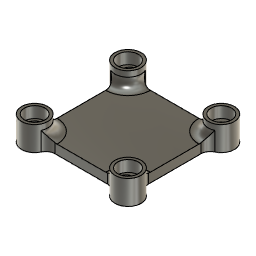
base (Autodesk Fusion 360 design; units mm, degrees)
Autodesk Fusion 360 part; units mm, degrees
sketch "Sketch1" plane through (0, 0, 0) normal (0, 0, 1) x (1, 0, 0)
  line L0 (-25, 25) -> (25, 25) construction
  line L1 (25, 25) -> (25, -25) construction
  line L2 (25, -25) -> (-25, -25) construction
  line L3 (-25, -25) -> (-25, 25) construction
  circle A0 centre (-25, 25) radius 7
  circle A1 centre (25, 25) radius 3.25
  circle A2 centre (25, -25) radius 7
  circle A3 centre (-25, -25) radius 4
  circle A4 centre (-25, -25) radius 7
  circle A5 centre (25, 25) radius 7
  line L4 (-28.25, 26) -> (-28.25, 24)
  arc A6 (-28.25, 24) -> (-21.75, 24) centre (-25, 24) ccw
  line L5 (-21.75, 24) -> (-21.75, 26)
  arc A7 (-21.75, 26) -> (-28.25, 26) centre (-25, 26) ccw
  line L6 (-25, 26) -> (-25, 24) construction
  line L7 (24, -28.25) -> (26, -28.25)
  arc A8 (26, -28.25) -> (26, -21.75) centre (26, -25) ccw
  line L8 (26, -21.75) -> (24, -21.75)
  arc A9 (24, -21.75) -> (24, -28.25) centre (24, -25) ccw
  line L9 (24, -25) -> (26, -25) construction
  line L10 (-18, 25) -> (18, 25)
  line L11 (25, 18) -> (25, -18)
  line L12 (18, -25) -> (-18, -25)
  line L13 (-25, -18) -> (-25, 18)
  circle A10 centre (-25, 25) radius 5.5
  circle A11 centre (25, 25) radius 5.5
  circle A12 centre (-25, -25) radius 5.5
  circle A13 centre (25, -25) radius 5.5
  line L14 (-7, 10) -> (-3, 10)
  line L15 (-3, 10) -> (-3, -10)
  line L16 (-3, -10) -> (-7, -10)
  line L17 (-7, -10) -> (-7, 10)
  line L18 (3, 10) -> (7, 10)
  line L19 (7, 10) -> (7, -10)
  line L20 (7, -10) -> (3, -10)
  line L21 (3, -10) -> (3, 10)
  point P0 (-25, 25)
  point P1 (25, -25)
  dimension "d1" = 50
  dimension "d2" = 50
  dimension "d3" = 25
  dimension "d4" = 25
  dimension "d5" = 6.5
  dimension "d6" = 14
  dimension "d7" = 8
  dimension "d8" = 14
  dimension "d9" = 14
  dimension "d10" = 14
  dimension "d11" = 6.5
  dimension "d12" = 2
  dimension "d13" = 6.5
  dimension "d14" = 2
  dimension "d17" = 11
  dimension "d18" = 11
  dimension "d19" = 11
  dimension "d20" = 11
  dimension "d27" = 3
  dimension "d28" = 3
  dimension "d29" = 4
  dimension "d30" = 4
  dimension "d31" = 20
  dimension "d32" = 20
  dimension "d33" = 10
  dimension "d34" = 10
  constraint horizontal L0
  constraint vertical L1
  constraint horizontal L2
  constraint vertical L3
  constraint coincident P0 L0.start
  constraint coincident L0.end L1.start
  constraint coincident P1 L1.end
  constraint coincident L2.end L3.start
  constraint concentric A3 A4
  constraint concentric A1 A5
  constraint tangent L4 A6
  constraint tangent A6 L5
  constraint parallel L4 L5
  constraint tangent L5 A7
  constraint tangent L4 A7
  constraint coincident L3 A6.centre
  constraint perpendicular L0 L6
  constraint midpoint L6 P0
  constraint tangent L7 A8
  constraint tangent A8 L8
  constraint parallel L7 L8
  constraint tangent L8 A9
  constraint tangent L7 A9
  constraint perpendicular L1 L9
  constraint midpoint L9 P1
  constraint coincident A0 L10.start
  constraint coincident L0 L10.start
  constraint coincident A5 L10.end
  constraint coincident L0 L10.end
  constraint coincident L1 L11.start
  constraint coincident A5 L11.start
  constraint coincident A2 L11.end
  constraint coincident L1 L11.end
  constraint coincident A2 L12.start
  constraint coincident L2 L12.start
  constraint coincident A4 L12.end
  constraint coincident L2 L12.end
  constraint coincident A4 L13.start
  constraint coincident L3 L13.start
  constraint coincident L3 L13.end
  constraint coincident A0 L13.end
  constraint concentric A5 A11
  constraint concentric A4 A12
  constraint horizontal L14
  constraint vertical L15
  constraint horizontal L16
  constraint vertical L17
  constraint horizontal L18
  constraint vertical L19
  constraint horizontal L20
  constraint vertical L21
  measures "d1" distance of P0 L0.end
  measures "d2" distance of L0.end P1
  measures "d3" distance of origin L0
  measures "d4" distance of origin L1
  measures "d5" diameter of A1
  measures "d6" diameter of A0
  measures "d7" diameter of A3
  measures "d8" diameter of A2
  measures "d9" diameter of A4
  measures "d10" diameter of A5
  measures "d11" diameter of A6
  measures "d12" distance of A7.centre A6.centre
  measures "d13" diameter of A8
  measures "d14" distance of A9.centre A8.centre
  measures "d17" diameter of A10
  measures "d18" diameter of A11
  measures "d19" diameter of A12
  measures "d20" diameter of A13
  measures "d27" distance of origin L15
  measures "d28" distance of origin L21
  measures "d29" distance of L19 L21
  measures "d30" distance of L15 L17
  measures "d31" distance of L18 L20
  measures "d32" distance of L14 L16
  measures "d33" distance of origin L14
  measures "d34" distance of origin L18
extrude "Extrude1" add sketch "Sketch1" along normal blind 5 contours A0 | A0 A2 A4 A5 L10 L11 L12 L13 | A5 | A4 | A2 | A10 | A11 | A12 | A13 | L14 L15 L16 L17 | L18 L19 L20 L21
extrude "Extrude2" add sketch "Sketch1" along normal blind 7 contours A10 | A11 | A12 | A13
extrude "Extrude3" add sketch "Sketch1" along normal blind 13 contours A0 | A5 | A4 | A2
fillet "Fillet1" radius 5 12 edges at (-20.0503, 20.0503, 5) (20.0503, 20.0503, 5) (-20.0503, -20.0503, 5) (20.0503, -20.0503, 5) (25, 18, 2.5) (-18, -25, 2.5) (-25, -18, 2.5) (18, -25, 2.5) (25, -18, 2.5) (-25, 18, 2.5) (-18, 25, 2.5) (18, 25, 2.5)
